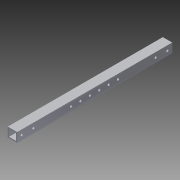
# Autodesk Inventor part: Chassis V1.500 Part7
Saved by Autodesk Inventor 2013 (Build 170138000, 138)
## iProperties
Created: 2013-01-18
Part Number: Chassis V1.500 Part7
Material: Aluminum 6061
Document SubType Name: Modeling
Designer: Moses
Mass: 314.683 g
Surface Area: 750.278 cm^2
Volume: 116.119 cm^3
Density: 2.71 g/cm^3
Author: Moses
Autodesk Inventor part; units mm, degrees
ref_plane "YZ Plane" through (0, 0, 0) normal (1, 0, 0) x (0, 1, 0)
ref_plane "XZ Plane" through (0, 0, 0) normal (0, 1, 0) x (-1, 0, 0)
ref_plane "XY Plane" through (0, 0, 0) normal (0, 0, 1) x (1, 0, 0)
sketch "Sketch1" plane through (0, 0, 0) normal (0, 0, 1) x (1, 0, 0)
  line L0 (0, 0) -> (25.4, 0)
  line L1 (25.4, 0) -> (25.4, 25.4)
  line L2 (25.4, 25.4) -> (0, 25.4)
  line L3 (0, 25.4) -> (0, 0)
  line L4 (3.175, 22.225) -> (22.225, 22.225)
  line L5 (22.225, 22.225) -> (22.225, 3.175)
  line L6 (22.225, 3.175) -> (3.175, 3.175)
  line L7 (3.175, 3.175) -> (3.175, 22.225)
  dimension "d0" = 25.4
  dimension "d1" = 25.4
  dimension "d2" = 3.175
  constraints: 16 end point, 4 parallel, 2 perpendicular, 1 horizontal, 3 other
  measures "d0" distance of L2.end L1.end
  measures "d1" distance of L1.end L0.end
  measures "d2" distance between parallel lines of L1 L5
extrude "Extrusion1" add sketch "Sketch1" along normal blind 419.1
sketch "Sketch2" plane through (25.4, 0, 0) normal (1, 0, 0) x (0, 0, -1)
  line L0 (-419.1, 0) -> (-419.1, 25.4) projected
  line L1 (0, 0) -> (-419.1, 0) projected
  line L2 (-419.1, 12.7) -> (-400.05, 12.7) construction
  circle A0 centre (-400.05, 12.7) radius 3.302 construction
  circle A1 centre (-374.65, 12.7) radius 3.302
  circle A2 centre (-349.25, 12.7) radius 3.302
  circle A3 centre (-323.85, 12.7) radius 3.302
  circle A4 centre (-298.45, 12.7) radius 3.302
  circle A5 centre (-273.05, 12.7) radius 3.302
  circle A6 centre (-247.65, 12.7) radius 3.302
  circle A7 centre (-222.25, 12.7) radius 3.302
  circle A8 centre (-196.85, 12.7) radius 3.302
  circle A9 centre (-171.45, 12.7) radius 3.302
  circle A10 centre (-146.05, 12.7) radius 3.302
  circle A11 centre (-120.65, 12.7) radius 3.302
  circle A12 centre (-95.25, 12.7) radius 3.302
  circle A13 centre (-69.85, 12.7) radius 3.302
  circle A14 centre (-44.45, 12.7) radius 3.302
  circle A15 centre (-19.05, 12.7) radius 3.302 construction
  line L3 (0, 0) -> (0, 25.4) projected
  circle A16 centre (-406.4, 12.7) radius 3.302
  circle A17 centre (-12.7, 12.7) radius 3.302
  line L4 (-12.7, 12.7) -> (0, 12.7) construction
  dimension "d5" = 19.05
  dimension "d7" = 6.604
  dimension "d10" = 419.1
  dimension "d13" = 25.4
  dimension "d18" = 19.05
  dimension "d19" = 12.7
  dimension "d20" = 6.604
  dimension "d21" = 6.604
  dimension "d22" = 12.7
  constraints: 18 centre point, 4 end point, 2 horizontal, 2 midpoint, 1 coincident, 1 parallel, 1 point on line, 30 other
  measures "d5" distance of L2.start L2.end
  measures "d7" diameter of A0
  measures "d10" distance of L3.end L0.end
  measures "d13" distance of A0.centre A1.centre
  measures "d18" distance from line of L3 A15.centre
  measures "d19" distance of L4.start L4.end
  measures "d20" diameter of A17
  measures "d21" diameter of A16
  measures "d22" distance from line of L0 A16.centre
extrude "Extrusion2" cut sketch "Sketch2" against normal through all contours A1 | A5 | A6 | A7 | A8 | A9 | A10 | A14 | A16 | A17
equation "\"d13\" = -0.133333 * d5 + 0.0666667 * d10"
equation "\"d20\" = d7"
equation "\"d21\" = d7"
equation "\"d22\" = d19"
body "Solid1"
